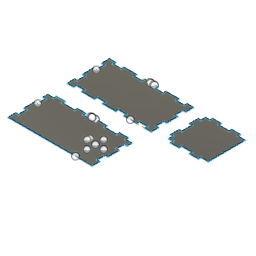
marvis_container v7 (Autodesk Fusion 360 design; units mm, degrees)
Autodesk Fusion 360 part; units mm, degrees
sketch "Sketch2" plane through (0, 0, 0) normal (0, 0, 1) x (1, 0, 0)
  line L0 (-41.35, 47.7316) -> (-42, 47.7316)
  line L1 (-107.0217, 47.7316) -> (-107.0217, 41.3816)
  line L2 (-107.0217, 41.3816) -> (-127.0217, 41.3816)
  line L3 (-127.0217, 41.3816) -> (-127.0217, 47.7316)
  line L4 (-44.9549, 47.7316) -> (-43, 47.7316)
  line L5 (-35.9147, 47.7316) -> (-33.6547, 47.7316)
  line L6 (-57.2038, 47.7316) -> (-57.2038, 41.3816)
  line L7 (-57.2038, 41.3816) -> (-77.2038, 41.3816)
  line L8 (-77.2038, 41.3816) -> (-77.2038, 47.7316)
  line L9 (-6.4037, 47.7316) -> (-6.4037, 41.3816)
  line L10 (-6.4037, 41.3816) -> (-26.4037, 41.3816)
  line L11 (-26.4037, 41.3816) -> (-26.4037, 47.7316)
  line L12 (43.8867, 47.7316) -> (43.8867, 41.3816)
  line L13 (43.8867, 41.3816) -> (23.8867, 41.3816)
  line L14 (23.8867, 41.3816) -> (23.8867, 47.7316)
  line L15 (58.65, -52.2684) -> (8.65, -52.2684) construction
  line L16 (-127.0217, -45.9184) -> (-127.0217, -52.2684)
  line L17 (-107.0217, -45.9184) -> (-127.0217, -45.9184)
  line L18 (-107.0217, -52.2684) -> (-107.0217, -45.9184)
  line L19 (-77.2038, -45.9184) -> (-77.2038, -52.2684)
  line L20 (-57.2038, -45.9184) -> (-77.2038, -45.9184)
  line L21 (-57.2038, -52.2684) -> (-57.2038, -45.9184)
  line L22 (-26.4037, -45.9184) -> (-26.4037, -52.2684)
  line L23 (-6.4037, -45.9184) -> (-26.4037, -45.9184)
  line L24 (-6.4037, -52.2684) -> (-6.4037, -45.9184)
  line L25 (23.8867, -45.9184) -> (23.8867, -52.2684)
  line L26 (43.8867, -45.9184) -> (23.8867, -45.9184)
  line L27 (43.8867, -52.2684) -> (43.8867, -45.9184)
  line L28 (-141.35, 30) -> (-135, 30)
  line L29 (-135, 30) -> (-135, 10)
  line L30 (-135, 10) -> (-141.35, 10)
  line L31 (-141.35, -15.6117) -> (-135, -15.6117)
  line L32 (-135, -15.6117) -> (-135, -35.6117)
  line L33 (-135, -35.6117) -> (-141.35, -35.6117)
  line L34 (58.65, 30) -> (52.3, 30)
  line L35 (52.3, 30) -> (52.3, 10)
  line L36 (52.3, 10) -> (58.65, 10)
  line L37 (58.65, -15.6117) -> (52.3, -15.6117)
  line L38 (52.3, -15.6117) -> (52.3, -35.6117)
  line L39 (52.3, -35.6117) -> (58.65, -35.6117)
  line L40 (-6.4037, -93.403) -> (-6.4037, -99.753)
  line L41 (-134.9998, -130) -> (-141.3497, -130)
  line L42 (-141.3498, -110) -> (-134.9998, -110)
  line L43 (52.3002, -110) -> (52.3002, -130)
  line L44 (-77.2027, -99.753) -> (-77.2027, -93.403)
  line L45 (-134.9998, -155.931) -> (-134.9998, -175.931)
  line L46 (-77.2027, -93.403) -> (-57.2027, -93.403)
  line L47 (-141.3498, -155.931) -> (-134.9998, -155.931)
  line L48 (52.3002, -130) -> (58.6501, -130)
  line L49 (23.8864, -93.403) -> (43.8864, -93.403)
  line L50 (-26.4037, -99.753) -> (-26.4037, -93.403)
  line L51 (-107.0217, -93.403) -> (-107.0217, -99.753)
  line L52 (52.3002, -155.931) -> (52.3002, -175.931)
  line L53 (-134.9998, -175.931) -> (-141.3498, -175.931)
  line L54 (-127.0217, -99.753) -> (-127.0217, -93.403)
  line L55 (23.8864, -99.753) -> (23.8864, -93.403)
  line L56 (-127.0217, -93.403) -> (-107.0217, -93.403)
  line L57 (-41.3498, -93.403) -> (-42, -93.403)
  line L58 (-35.9147, -93.403) -> (-33.6547, -93.403)
  line L59 (-134.9998, -110) -> (-134.9998, -130)
  line L60 (58.6502, -193.403) -> (18.6502, -193.403) construction
  line L61 (-44.9549, -93.403) -> (-43, -93.403)
  line L62 (58.6502, -110) -> (52.3002, -110)
  line L63 (58.6502, -155.931) -> (52.3002, -155.931)
  line L64 (43.8864, -93.403) -> (43.8864, -99.753)
  line L65 (-26.4037, -93.403) -> (-6.4037, -93.403)
  line L66 (-57.2027, -93.403) -> (-57.2027, -99.753)
  line L67 (52.3002, -175.931) -> (58.6502, -175.931)
  line L68 (-127.0217, -99.753) -> (-141.3498, -99.753)
  line L69 (-127.0217, -93.403) -> (-107.0217, -93.403)
  line L70 (-107.0217, -99.753) -> (-77.2027, -99.753)
  line L71 (-57.2027, -99.753) -> (-26.4037, -99.753)
  line L72 (-6.4037, -99.753) -> (23.8864, -99.753)
  line L73 (43.8864, -99.753) -> (58.6502, -99.753)
  line L74 (-141.3498, -193.403) -> (58.6502, -193.403)
  line L75 (188.368, 41.3816) -> (188.368, -45.9184)
  line L76 (94.718, 30) -> (88.368, 30)
  line L77 (88.368, 30) -> (88.368, 10)
  line L78 (88.368, 10) -> (94.718, 10)
  line L79 (94.718, -15.6117) -> (88.368, -15.6117)
  line L80 (88.368, -15.6117) -> (88.368, -35.6117)
  line L81 (88.368, -35.6117) -> (94.718, -35.6117)
  line L82 (94.718, -45.9184) -> (104.965, -45.9184) construction
  line L83 (124.965, -45.9184) -> (124.965, -52.2684)
  line L84 (124.965, -52.2684) -> (104.965, -52.2684)
  line L85 (104.965, -52.2684) -> (104.965, -45.9184)
  line L86 (188.368, -45.9184) -> (170.896, -45.9184)
  line L87 (150.896, -45.9184) -> (150.896, -52.2684)
  line L88 (150.896, -52.2684) -> (170.896, -52.2684)
  line L89 (170.896, -52.2684) -> (170.896, -45.9184)
  line L90 (104.965, 47.7316) -> (104.965, 41.3816)
  line L91 (124.965, 47.7316) -> (104.965, 47.7316)
  line L92 (124.965, 41.3816) -> (124.965, 47.7316)
  line L93 (150.896, 41.3816) -> (150.896, 47.7316)
  line L94 (150.896, 47.7316) -> (170.896, 47.7316)
  line L95 (170.896, 47.7316) -> (170.896, 41.3816)
  line L96 (58.6502, -99.753) -> (58.6502, -110)
  line L97 (58.6502, -110) -> (52.3002, -110)
  line L98 (58.6502, -193.403) -> (58.6502, -175.931)
  line L99 (58.6502, -155.931) -> (58.6501, -130)
  line L100 (-141.3498, -99.753) -> (-141.3498, -110)
  line L101 (-141.3497, -130) -> (-141.3498, -155.931)
  line L102 (-141.3498, -175.931) -> (-141.3498, -193.403)
  line L103 (-127.0217, 47.7316) -> (-135, 47.7316)
  line L104 (-107.0217, 47.7316) -> (-77.2038, 47.7316)
  line L105 (-57.2038, 47.7316) -> (-26.4037, 47.7316)
  line L106 (-6.4037, 47.7316) -> (23.8867, 47.7316)
  line L107 (-135, 47.7316) -> (-141.35, 47.7316)
  line L108 (-141.35, 47.7316) -> (-141.35, 30)
  line L109 (-141.35, 10) -> (-141.35, -15.6117)
  line L110 (-141.35, -35.6117) -> (-141.35, -52.2684)
  line L111 (-141.35, -52.2684) -> (-127.0217, -52.2684)
  line L112 (-107.0217, -52.2684) -> (-77.2038, -52.2684)
  line L113 (-57.2038, -52.2684) -> (-26.4037, -52.2684)
  line L114 (-6.4037, -52.2684) -> (23.8867, -52.2684)
  line L115 (43.8867, -52.2684) -> (58.65, -52.2684)
  line L116 (58.65, -35.6117) -> (58.65, -52.2684)
  line L117 (58.65, -15.6117) -> (58.65, 10)
  line L118 (43.8867, 47.7316) -> (58.65, 47.7316)
  line L119 (58.65, 47.7316) -> (58.65, 30)
  line L120 (104.965, 41.3816) -> (94.718, 41.3816)
  line L121 (94.718, 41.3816) -> (94.718, 30)
  line L122 (94.718, 10) -> (94.718, -15.6117)
  line L123 (94.718, -35.6117) -> (94.718, -45.9184)
  line L124 (94.718, -45.9184) -> (104.965, -45.9184)
  line L125 (124.965, -45.9184) -> (150.896, -45.9184)
  line L126 (188.368, 41.3816) -> (170.896, 41.3816)
  line L127 (150.896, 41.3816) -> (124.965, 41.3816)
  circle A0 centre (18.6502, -145.903) radius 2.35
  circle A1 centre (-1.3498, -145.903) radius 2.35
  circle A2 centre (18.6502, -125.903) radius 2.35
  circle A3 centre (38.6502, -145.903) radius 2.35
  circle A4 centre (18.6502, -165.903) radius 2.35
  point P0 (-135, 10)
  point P1 (-135, -130)
  point P2 (0, -140)
  dimension "d13" = 6.35
  dimension "d14" = 20
  dimension "d15" = 20
  dimension "d16" = 6.35
  dimension "d17" = 20
  dimension "d18" = 6.35
  dimension "d19" = 20
  dimension "d20" = 6.35
  dimension "d21" = 50
  dimension "d22" = 6.35
  dimension "d23" = 20
  dimension "d24" = 6.35
  dimension "d25" = 20
  dimension "d28" = 6.35
  dimension "d29" = 20
  dimension "d30" = 20
  dimension "d31" = 6.35
  dimension "d32" = 20
  dimension "d33" = 6.35
  dimension "d34" = 20
  dimension "d35" = 6.35
  dimension "d36" = 40
  dimension "d37" = 6.35
  dimension "d38" = 20
  dimension "d39" = 6.35
  dimension "d40" = 20
  dimension "d43" = 6.35
  dimension "d44" = 20
  dimension "d45" = 6.35
  dimension "d46" = 20
  dimension "d47" = 10.247
  dimension "d48" = 10.247
  dimension "d49" = 20
  dimension "d50" = 6.35
  dimension "d51" = 10.247
  dimension "d52" = 17.472
  dimension "d53" = 17.472
  dimension "d54" = 17.472
  dimension "d55" = 20
  dimension "d56" = 6.35
  dimension "d57" = 100
  dimension "d62" = 47.5
  dimension "d63" = 4.7
  dimension "d64" = 20
  dimension "d65" = 20
  dimension "d66" = 20
  dimension "d67" = 20
  dimension "d68" = 4.7
  dimension "d69" = 4.7
  dimension "d70" = 4.7
  dimension "d71" = 4.7
  constraint horizontal L0
  constraint vertical L1
  constraint horizontal L2
  constraint vertical L3
  constraint horizontal L4
  constraint horizontal L5
  constraint vertical L6
  constraint horizontal L7
  constraint vertical L8
  constraint vertical L9
  constraint horizontal L10
  constraint vertical L11
  constraint vertical L12
  constraint horizontal L13
  constraint vertical L14
  constraint horizontal L28
  constraint vertical L29
  constraint horizontal L30
  constraint horizontal L31
  constraint vertical L32
  constraint horizontal L33
  constraint horizontal L57
  constraint horizontal L56
  constraint vertical L51
  constraint vertical L54
  constraint horizontal L61
  constraint horizontal L58
  constraint horizontal L46
  constraint vertical L66
  constraint vertical L44
  constraint horizontal L65
  constraint vertical L40
  constraint vertical L50
  constraint horizontal L49
  constraint vertical L64
  constraint vertical L55
  constraint horizontal L42
  constraint vertical L59
  constraint horizontal L41
  constraint horizontal L47
  constraint vertical L45
  constraint horizontal L53
  constraint vertical L75
  constraint horizontal L76
  constraint vertical L77
  constraint horizontal L78
  constraint horizontal L79
  constraint vertical L80
  constraint horizontal L81
  constraint vertical L83
  constraint horizontal L84
  constraint vertical L85
  constraint perpendicular L75 L86
  constraint vertical L87
  constraint horizontal L88
  constraint vertical L89
  constraint perpendicular L67 L98
  constraint perpendicular L42 L100
  constraint perpendicular L74 L102
  constraint perpendicular L3 L103
  constraint perpendicular L8 L104
  constraint perpendicular L11 L105
  constraint perpendicular L14 L106
  constraint perpendicular L28 L108
  constraint perpendicular L31 L109
  constraint perpendicular L33 L110
  constraint perpendicular L16 L111
  constraint perpendicular L27 L115
  constraint perpendicular L15 L116
  constraint perpendicular L12 L118
  constraint perpendicular L34 L119
  constraint perpendicular L90 L120
  constraint perpendicular L76 L121
  constraint perpendicular L79 L122
  constraint perpendicular L82 L123
  constraint perpendicular L85 L124
  constraint perpendicular L87 L125
  constraint perpendicular L95 L126
  constraint perpendicular L92 L127
  measures "d13" distance of L3.end L2.end
  measures "d14" distance of L3.end L1.start
  measures "d15" distance of L8.end L6.start
  measures "d16" distance of L8.end L7.end
  measures "d17" distance of L11.end L9.start
  measures "d18" distance of L11.end L10.end
  measures "d19" distance of L14.end L12.start
  measures "d20" distance of L14.end L13.end
  measures "d21" distance of L15.start L15.end
  measures "d22" distance of L28.start L28.end
  measures "d23" distance of L28.start L30.end
  measures "d24" distance of L31.start L31.end
  measures "d25" distance of L31.start L33.end
  measures "d28" distance of L54.end L54.start
  measures "d29" distance of L51.start L54.end
  measures "d30" distance of L44.end L46.end
  measures "d31" distance of L44.start L44.end
  measures "d32" distance of L40.start L50.end
  measures "d33" distance of L50.start L50.end
  measures "d34" distance of L49.end L49.start
  measures "d35" distance of L49.start L55.start
  measures "d36" distance of L60.end L60.start
  measures "d37" distance of L42.start L42.end
  measures "d38" distance of L42.start L41.end
  measures "d39" distance of L47.start L45.start
  measures "d40" distance of L47.start L53.end
  measures "d43" distance of L76.start L76.end
  measures "d44" distance of L76.start L78.end
  measures "d45" distance of L79.start L79.end
  measures "d46" distance of L79.start L81.end
  measures "d47" distance of L62.start L73.end
  measures "d48" distance of L82.start L82.end
  measures "d49" distance of L82.end L83.start
  measures "d50" distance of L82.end L84.end
  measures "d51" distance of L42.start L68.end
  measures "d52" vertical distance of L67.end L60.start
  measures "d53" distance of L53.end L74.start
  measures "d54" distance of L75.end L86.end
  measures "d55" distance of L86.end L87.start
  measures "d56" distance of L86.end L88.end
  measures "d57" distance of L49.end L60
  measures "d62" distance of L60.end A0.centre
  measures "d63" diameter of A0
  measures "d64" distance of A0.centre A1.centre
  measures "d65" distance of A0.centre A3.centre
  measures "d66" distance of A0.centre A2.centre
  measures "d67" distance of A0.centre A4.centre
  measures "d68" diameter of A1
  measures "d69" diameter of A2
  measures "d70" diameter of A3
  measures "d71" diameter of A4
extrude "Extrude1" add sketch "Sketch2" along normal blind 1 contours L0 L1 L2 L3 L4 L5 L6 L7 L8 L9 L10 L11 L12 L13 L14 L16 L17 L18 L19 L20 L21 L22 L23 L24 L25 L26 L27 L28 L29 L30 L31 L32 L33 L34 L35 L36 L37 L38 L39 L103 L104 L105 L106 L107 L108 L109 L110 L111 L112 L113 L114 L115 L116 L117 L118 L119 makes body 1
extrude "Extrude2" add sketch "Sketch2" along normal blind 1 separate body contours L40 L41 L42 L43 L44 L45 L46 L47 L48 L49 L50 L51 L52 L53 L54 L55 L56 L59 L62 L63 L64 L65 L66 L67 L68 L69 L70 L71 L72 L73 L74 L96 L97 L98 L99 L100 L101 L102 | L75 L76 L77 L78 L79 L80 L81 L83 L84 L85 L86 L87 L88 L89 L90 L91 L92 L93 L94 L95 L120 L121 L122 L123 L124 L125 L126 L127 | A0 | A1 | A2 | A3 | A4 makes body 2 at (132.17, 1.8211, 0) makes body 3 at (-36.3678, -150.5383, 0)
equation "width = 200 mm"
equation "length = 100 mm"
equation "height = 100 mm"
equation "thickness = 6.35 mm"
equation "d13 = thickness"
equation "d16 = thickness"
equation "d18 = thickness"
equation "d20 = thickness"
equation "d22 = thickness"
equation "d24 = thickness"
equation "d28 = thickness"
equation "d31 = thickness"
equation "d33 = thickness"
equation "d35 = thickness"
equation "d37 = thickness"
equation "d39 = thickness"
equation "d43 = thickness"
equation "d45 = thickness"
equation "d50 = thickness"
equation "d56 = thickness"
